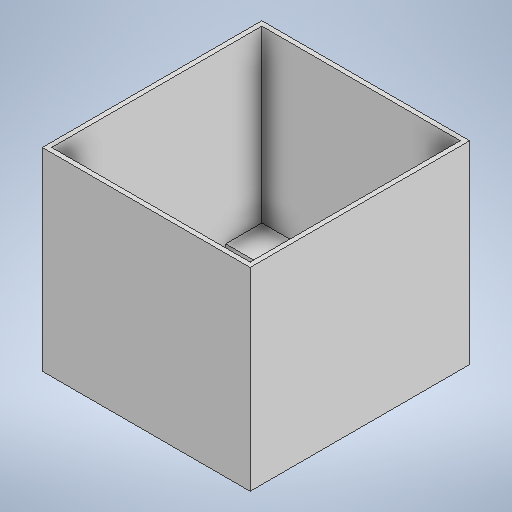
# Autodesk Inventor part: Arduino_case
Saved by Autodesk Inventor 2025.2 (Build 292293000, 293)
## iProperties
Created: 2025-09-19
Part Number: Arduino_case
Material: Generic
Document SubType Name: Modeling
Designer: TSO
Density: 1 g/cm^3
Appearance: Default
Author: TSO
Autodesk Inventor part; units mm, degrees
ref_plane "YZ Plane" through (0, 0, 0) normal (1, 0, 0) x (0, 1, 0)
ref_plane "XZ Plane" through (0, 0, 0) normal (0, 1, 0) x (-1, 0, 0)
ref_plane "XY Plane" through (0, 0, 0) normal (0, 0, 1) x (1, 0, 0)
sketch "Sketch1" plane through (0, 0, 0) normal (0, 1, 0) x (-1, 0, 0)
  line L0 (0, 0) -> (89, 0)
  line L1 (89, 0) -> (89, -94)
  line L2 (89, -94) -> (0, -94)
  line L3 (0, -94) -> (0, 0)
  dimension "d0" = 89
  dimension "d1" = 94
  constraints: 8 end point, 2 parallel, 1 horizontal, 1 perpendicular
  measures "d0" distance of L1.end L2.end
  measures "d1" distance of L0.end L1.end
extrude "Extrusion1" add sketch "Sketch1" along normal blind 83
sketch "Sketch2" plane through (0, 83, 0) normal (0, 1, 0) x (1, 0, 0)
  line L0 (0, 0) -> (0, 2) construction
  line L1 (0, 0) -> (0, 94) projected
  line L2 (0, 2) -> (-2, 2) construction
  line L3 (-2, 2) -> (-87, 2)
  line L4 (-87, 2) -> (-87, 92)
  line L5 (-87, 92) -> (-2, 92)
  line L6 (-2, 92) -> (-2, 2)
  dimension "d4" = 2
  dimension "d5" = 2
  dimension "d6" = 85
  dimension "d7" = 90
  constraints: 12 end point, 2 horizontal, 2 parallel, 1 perpendicular, 1 point on line
  measures "d4" distance of L0.start L0.end
  measures "d5" distance of L0.end L2.end
  measures "d6" distance of L4.end L5.end
  measures "d7" distance of L3.end L4.end
extrude "Extrusion2" cut sketch "Sketch2" against normal blind 81
sketch "Sketch3" plane through (0, 2, 0) normal (0, 1, 0) x (1, 0, 0)
  line L0 (-87, 2) -> (-87, 92) projected
  line L1 (-87, 2) -> (-76, 2)
  line L2 (-2, 2) -> (-87, 2) projected
  line L3 (-76, 2) -> (-17, 2)
  line L4 (-87, 92) -> (-2, 92) projected
  line L5 (-76, 2) -> (-87, 2)
  line L6 (-87, 2) -> (-87, 92)
  line L7 (-87, 92) -> (-76, 92)
  line L8 (-2, 92) -> (-2, 2) projected
  line L9 (-17, 2) -> (-2, 2)
  line L10 (-2, 2) -> (-2, 92)
  line L11 (-2, 92) -> (-17, 92)
  line L12 (-87, 2) -> (-87, 17.5)
  line L13 (-87, 17.5) -> (-87, 76.5)
  line L14 (-87, 17.5) -> (-2, 17.5)
  line L15 (-2, 17.5) -> (-2, 2)
  line L16 (-2, 2) -> (-87, 2)
  line L17 (-87, 2) -> (-87, 17.5)
  line L18 (-87, 76.5) -> (-2, 76.5)
  line L19 (-2, 76.5) -> (-2, 92)
  line L20 (-2, 92) -> (-87, 92)
  line L21 (-87, 92) -> (-87, 76.5)
  point P0 (0, 0)
  point P1 (-2, 76.5)
  point P2 (-2, 17.5)
  dimension "d26" = 15.5
  dimension "d27" = 59
  constraints: 36 end point, 6 parallel, 4 horizontal, 4 perpendicular, 4 point on line
  measures "d26" distance of L5.end L12.end
  measures "d27" distance of L12.end L13.end
extrude "Extrusion3" add sketch "Sketch3" along normal blind 8 contours L0 L14 L8 L2 L1 | L0 L4 L8 L18
sketch "Sketch4" plane through (0, 2, 0) normal (0, 1, 0) x (1, 0, 0)
  line L0 (-46.5, 2) -> (43.5, 2) construction
  line L1 (-2, 17.5) -> (-87, 17.5) projected
  line L2 (-2, 17.5) -> (-6.5, 17.5)
  line L3 (-6.5, 17.5) -> (-6.5, 22.5)
  line L4 (-6.5, 22.5) -> (-2, 22.5)
  line L5 (-2, 22.5) -> (-2, 17.5)
  line L6 (-2, 76.5) -> (-2, 17.5) projected
  line L7 (-2, 76.5) -> (-6.5, 76.5)
  line L8 (-6.5, 76.5) -> (-6.5, 66.5)
  line L9 (-6.5, 66.5) -> (-2, 66.5)
  line L10 (-2, 66.5) -> (-2, 76.5)
  line L11 (-87, 17.5) -> (-81.2, 17.5)
  line L12 (-81.2, 17.5) -> (-81.2, 21.7)
  line L13 (-81.2, 21.7) -> (-87, 21.7)
  line L14 (-87, 21.7) -> (-87, 17.5)
  circle A0 centre (-81.2, 21.7) radius 1.35
  line L15 (-87, 17.5) -> (-87, 76.5) projected
  line L16 (-87, 47) -> (-2, 47) construction
  circle A1 centre (-81.2, 72.3) radius 1.35
  point P0 (-76, 2)
  dimension "d28" = 4.5
  dimension "d29" = 5
  dimension "d30" = 4.5
  dimension "d31" = 10
  dimension "d32" = 5.8
  dimension "d33" = 4.2
  dimension "d34" = 2.7
  constraints: 28 end point, 6 parallel, 4 horizontal, 3 perpendicular, 2 centre point, 2 midpoint, 1 coincident, 1 symmetric about line, 1 other
  measures "d28" distance of L3.end L4.end
  measures "d29" distance of L2.end L3.end
  measures "d30" distance of L9.end L8.end
  measures "d31" distance of L8.end L7.end
  measures "d32" distance of L13.end L12.end
  measures "d33" distance of L12.end L11.end
  measures "d34" diameter of A0
extrude "Extrusion4" add sketch "Sketch4" along normal blind 3 contours L1 L3 L4 L5 | A0 L13 L12 | L12 L13 A0 | L6 L9 L8 L7 | A1
sketch "Sketch6" plane through (-89, 0, -94) normal (-1, 0, 0) x (0, 0, 1)
  line L0 (0, 0) -> (0, 83) projected
  line L1 (0, 0) -> (2, 0) construction
  line L2 (2, 0) -> (2, 2) construction
  line L3 (2, 2) -> (0, 2) construction
  line L4 (0, 2) -> (0, 0)
  line L5 (2, 2) -> (27.5, 2) construction
  line L6 (20.35, 2) -> (20.35, 5) projected
  line L7 (2, 2) -> (27.5, 2) construction
  line L8 (27.5, 2) -> (27.5, 8.8) construction
  line L9 (27.5, 2) -> (34.3, 2) construction
  line L10 (27.5, 8.8) -> (41.5, 8.8)
  line L11 (41.5, 8.8) -> (41.5, 14.8)
  line L12 (41.5, 14.8) -> (27.5, 14.8)
  line L13 (27.5, 14.8) -> (27.5, 8.8)
  line L14 (94, 0) -> (92, 0) construction
  line L15 (92, 0) -> (92, 2) construction
  line L16 (92, 2) -> (94, 2) construction
  line L17 (94, 2) -> (94, 0) construction
  line L18 (92, 2) -> (76.5, 2) construction
  line L19 (76.5, 2) -> (71.5, 2) construction
  line L20 (71.5, 2) -> (71.5, 10) construction
  line L21 (71.5, 10) -> (60.5, 10)
  line L22 (60.5, 10) -> (60.5, 23)
  line L23 (60.5, 23) -> (71.5, 23)
  line L24 (71.5, 23) -> (71.5, 10)
  dimension "d35" = 2
  dimension "d36" = 2
  dimension "d37" = 25.5
  dimension "d38" = 0
  dimension "d39" = 6.8
  dimension "d40" = 90
  dimension "d41" = 14
  dimension "d42" = 6
  dimension "d43" = 2
  dimension "d44" = 2
  dimension "d45" = 15.5
  dimension "d46" = 5
  dimension "d47" = 8
  dimension "d48" = 11
  dimension "d49" = 13
  constraints: 46 end point, 8 parallel, 7 horizontal, 6 perpendicular, 2 equal length, 1 point on line, 1 vertical
  measures "d35" distance of L3.end L2.end
  measures "d36" distance of L2.end L1.end
  measures "d37" distance of L2.end L5.end
  measures "d38" distance between parallel lines of L5 L7
  measures "d39" distance of L7.end L8.end
  measures "d40" angle of L9 L8
  measures "d41" distance of L12.end L11.end
  measures "d42" distance of L11.end L10.end
  measures "d43" distance of L15.end L16.end
  measures "d44" distance of L14.end L15.end
  measures "d45" distance of L15.end L18.end
  measures "d46" distance of L18.end L19.end
  measures "d47" distance of L19.end L20.end
  measures "d48" distance of L22.end L23.end
  measures "d49" distance of L21.end L22.end
extrude "Extrusion5" cut sketch "Sketch6" against normal up to surface (2 mm away)
body "Solid1"
